Autodesk Fusion 360 part; units mm, degrees
(part 3 of 3)
sketch "Sketch12" plane through (0, 0, 6) normal (0, 0, 1) x (-1, 0, 0)
  line L0 (-92.4617, 84.1384) -> (-86.7336, 92.5805)
  line L1 (-86.7336, 92.5805) -> (-82.7739, 89.3746)
  line L2 (-82.7739, 89.3746) -> (-92.4617, 84.1384)
  line L3 (-84.0126, 80.6229) -> (-80.1679, 87.2648)
  line L4 (-80.1679, 87.2648) -> (-76.1584, 84.0186)
  line L5 (-76.1584, 84.0186) -> (-84.0126, 80.6229)
  line L6 (-75.564, 76.5813) -> (-73.4538, 81.829)
  line L7 (-73.4538, 81.829) -> (-68.7023, 77.9821)
  line L8 (-68.7023, 77.9821) -> (-75.564, 76.5813)
  line L9 (-66.0187, 71.228) -> (-65.6021, 75.4722)
  line L10 (-65.6021, 75.4722) -> (-60.6844, 71.4907)
  line L11 (-60.6844, 71.4907) -> (-66.0187, 71.228)
  line L12 (-49.5335, 59.4079) -> (-45.3919, 59.1098)
  line L13 (-45.3919, 59.1098) -> (-45.0146, 55.4505)
  spline S0 degree 3 poles (-45.0146, 55.4505) (-46.4903, 56.8) (-47.9962, 58.1195) (-49.5335, 59.4079) knots 0.296583 0.296583 0.296583 0.296583 0.351349 0.351349 0.351349 0.351349
  line L14 (-37.9212, 53.0614) -> (-37.9212, 51.766)
  line L15 (-37.9212, 51.766) -> (-37.9212, 48.4975)
  spline S1 degree 3 poles (-37.9212, 48.4975) (-39.1883, 49.8271) (-40.4796, 51.1327) (-41.7959, 52.4137) knots 0.205807 0.205807 0.205807 0.205807 0.256159 0.256159 0.256159 0.256159
  line L16 (-41.7959, 52.4137) -> (-37.9212, 53.0614)
  line L17 (-35.1263, 45.4835) -> (-30.3557, 46.9362)
  line L18 (-30.3557, 46.9362) -> (-32.0809, 42.0059)
  spline S2 degree 3 poles (-32.0809, 42.0059) (-33.0798, 43.1811) (-34.0948, 44.3405) (-35.1263, 45.4835) knots 0.126094 0.126094 0.126094 0.126094 0.168261 0.168261 0.168261 0.168261
  spline S3 degree 3 poles (-26.1093, 34.5476) (-27.3076, 36.135) (-28.5305, 37.698) (-29.7792, 39.2354) knots 0.039267 0.039267 0.039267 0.039267 0.093303 0.093303 0.093303 0.093303
  line L19 (-29.7792, 39.2354) -> (-23.1969, 41.1404)
  line L20 (-23.1969, 41.1404) -> (-26.1093, 34.5476)
  line L21 (-27.7829, 47.0202) -> (-22.7358, 48.9312)
  line L22 (-22.7358, 48.9312) -> (-23.5672, 43.6191)
  line L23 (-23.5672, 43.6191) -> (-27.7829, 47.0202)
  line L24 (-35.0824, 52.9091) -> (-30.8262, 53.9269)
  line L25 (-30.8262, 53.9269) -> (-30.8262, 49.4754)
  line L26 (-30.8262, 49.4754) -> (-35.0824, 52.9091)
  line L27 (-42.6724, 59.0324) -> (-38.5427, 59.1325)
  line L28 (-38.5427, 59.1325) -> (-38.3359, 55.5339)
  line L29 (-38.3359, 55.5339) -> (-42.6724, 59.0324)
  line L30 (-53.3931, 70.682) -> (-57.6141, 71.0867)
  line L31 (-57.6141, 71.0867) -> (-58.1695, 74.9342)
  spline S4 degree 3 poles (-58.1695, 74.9342) (-57.6496, 74.4545) (-57.1267, 73.9777) (-56.6007, 73.5039) (-55.5434, 72.5513) (-54.4741, 71.6108) (-53.3931, 70.682) knots -0.519753 -0.519753 -0.519753 -0.519753 -0.5 -0.5 -0.5 -0.460292 -0.460292 -0.460292 -0.460292
  line L32 (-61.6594, 78.2411) -> (-66.3286, 78.1172)
  line L33 (-66.3286, 78.1172) -> (-66.0088, 82.615)
  spline S5 degree 3 poles (-66.0088, 82.615) (-64.5832, 81.1337) (-63.1337, 79.6754) (-61.6594, 78.2411) knots -0.622035 -0.622035 -0.622035 -0.622035 -0.564532 -0.564532 -0.564532 -0.564532
  line L34 (-68.7436, 85.5164) -> (-73.8681, 84.1998)
  line L35 (-73.8681, 84.1998) -> (-72.3108, 89.4858)
  spline S6 degree 3 poles (-72.3108, 89.4858) (-71.1388, 88.1462) (-69.95, 86.8228) (-68.7436, 85.5164) knots -0.708932 -0.708932 -0.708932 -0.708932 -0.659206 -0.659206 -0.659206 -0.659206
  line L36 (-74.6324, 92.1865) -> (-80.4342, 89.497)
  line L37 (-80.4342, 89.497) -> (-77.8281, 96.0622)
  spline S7 degree 3 poles (-77.8281, 96.0622) (-76.7771, 94.7566) (-75.7121, 93.4645) (-74.6324, 92.1865) knots -0.788777 -0.788777 -0.788777 -0.788777 -0.742083 -0.742083 -0.742083 -0.742083
  line L38 (-85.6123, 93.6745) -> (-78.9776, 97.5027)
  line L39 (-78.9776, 97.5027) -> (-81.7381, 90.5489)
  line L40 (-81.7381, 90.5489) -> (-85.6123, 93.6745)
  line L41 (-79.0459, 88.377) -> (-73.5557, 90.9221)
  line L42 (-73.5557, 90.9221) -> (-75.2158, 85.2871)
  line L43 (-75.2158, 85.2871) -> (-79.0459, 88.377)
  line L44 (-72.3151, 82.9469) -> (-67.5013, 84.1835)
  line L45 (-67.5013, 84.1835) -> (-67.8456, 79.3411)
  line L46 (-67.8456, 79.3411) -> (-72.3151, 82.9469)
  line L47 (-64.4078, 76.5676) -> (-60.0386, 76.6835)
  line L48 (-60.0386, 76.6835) -> (-59.4437, 72.5628)
  line L49 (-59.4437, 72.5628) -> (-64.4078, 76.5676)
  spline S8 degree 3 poles (-45.0116, 63.8871) (-43.5935, 62.8013) (-42.1585, 61.7326) (-40.7069, 60.6805) knots -0.360336 -0.360336 -0.360336 -0.360336 -0.310857 -0.310857 -0.310857 -0.310857
  line L50 (-40.7069, 60.6805) -> (-44.5984, 60.5862)
  line L51 (-44.5984, 60.5862) -> (-45.0116, 63.8871)
  line L52 (-32.6725, 55.1305) -> (-36.6553, 54.1781)
  line L53 (-36.6553, 54.1781) -> (-36.873, 57.9658)
  spline S9 degree 3 poles (-36.873, 57.9658) (-35.4867, 57.0067) (-34.0863, 56.0618) (-32.6725, 55.1305) knots -0.267714 -0.267714 -0.267714 -0.267714 -0.221358 -0.221358 -0.221358 -0.221358
  line L54 (-24.4898, 49.9779) -> (-29.2262, 48.1845)
  line L55 (-29.2262, 48.1845) -> (-29.2262, 52.9038)
  spline S10 degree 3 poles (-29.2262, 52.9038) (-27.6627, 51.913) (-26.0837, 50.9379) (-24.4898, 49.9779) knots -0.183976 -0.183976 -0.183976 -0.183976 -0.133479 -0.133479 -0.133479 -0.133479
  line L56 (-15.7266, 44.9303) -> (-22.1293, 42.4591)
  line L57 (-22.1293, 42.4591) -> (-21.2525, 48.0608)
  spline S11 degree 3 poles (-21.2525, 48.0608) (-19.8324, 47.2338) (-18.401, 46.4181) (-16.9588, 45.6135) (-16.549, 45.3849) (-16.1382, 45.1571) (-15.7266, 44.9303) knots -0.099506 -0.099506 -0.099506 -0.099506 -0.055069 -0.055069 -0.055069 -0.042441 -0.042441 -0.042441 -0.042441
  line L58 (-30.8842, 40.5813) -> (-29.0347, 45.8668)
  line L59 (-29.0347, 45.8668) -> (-24.7124, 42.3674)
  line L60 (-24.7124, 42.3674) -> (-30.8842, 40.5813)
  line L61 (-36.3212, 46.7922) -> (-36.3212, 51.766)
  line L62 (-36.3212, 51.766) -> (-31.8569, 48.1516)
  line L63 (-31.8569, 48.1516) -> (-36.3212, 46.7922)
  line L64 (-43.2354, 53.7952) -> (-43.6369, 57.6889)
  line L65 (-43.6369, 57.6889) -> (-39.5819, 54.4059)
  line L66 (-39.5819, 54.4059) -> (-43.2354, 53.7952)
  line L67 (-63.64, 69.7432) -> (-58.8192, 69.9806)
  line L68 (-58.8192, 69.9806) -> (-58.101, 66.0186)
  spline S12 degree 3 poles (-58.101, 66.0186) (-59.9089, 67.2995) (-61.7555, 68.5409) (-63.64, 69.7432) knots 0.44941 0.44941 0.44941 0.44941 0.509295 0.509295 0.509295 0.509295
  line L69 (-73.3235, 75.4057) -> (-67.0915, 76.678)
  line L70 (-67.0915, 76.678) -> (-67.5366, 72.1422)
  spline S13 degree 3 poles (-67.5366, 72.1422) (-69.4303, 73.2669) (-71.3596, 74.3545) (-73.3235, 75.4057) knots 0.550019 0.550019 0.550019 0.550019 0.608612 0.608612 0.608612 0.608612
  line L71 (-82.0425, 79.7315) -> (-74.7548, 82.8823)
  line L72 (-74.7548, 82.8823) -> (-76.996, 77.3086)
  spline S14 degree 3 poles (-76.996, 77.3086) (-77.9206, 77.7723) (-78.8524, 78.2283) (-79.7914, 78.6767) (-80.5375, 79.0329) (-81.2878, 79.3845) (-82.0425, 79.7315) knots 0.644744 0.644744 0.644744 0.644744 0.671746 0.671746 0.671746 0.693198 0.693198 0.693198 0.693198
  line L73 (-90.517, 83.3708) -> (-81.4267, 88.284)
  line L74 (-81.4267, 88.284) -> (-85.4862, 81.271)
  spline S15 degree 3 poles (-85.4862, 81.271) (-87.1438, 81.9913) (-88.821, 82.691) (-90.517, 83.3708) knots 0.725554 0.725554 0.725554 0.725554 0.77189 0.77189 0.77189 0.77189
  spline S16 degree 3 poles (-93.9955, 84.7275) (-96.255, 85.585) (-98.5463, 86.4092) (-100.8677, 87.202) knots 0.803334 0.803334 0.803334 0.803334 0.864159 0.864159 0.864159 0.864159
  line L75 (-100.8677, 87.202) -> (-87.9816, 93.5909)
  line L76 (-87.9816, 93.5909) -> (-93.9955, 84.7275)
  line L77 (22.7358, 48.9312) -> (27.7829, 47.0202)
  line L78 (27.7829, 47.0202) -> (23.5672, 43.6191)
  line L79 (23.5672, 43.6191) -> (22.7358, 48.9312)
  line L80 (30.8262, 53.9269) -> (35.0824, 52.9091)
  line L81 (35.0824, 52.9091) -> (30.8262, 49.4754)
  line L82 (30.8262, 49.4754) -> (30.8262, 53.9269)
  line L83 (38.5427, 59.1325) -> (42.6724, 59.0324)
  line L84 (42.6724, 59.0324) -> (38.3359, 55.5339)
  line L85 (38.3359, 55.5339) -> (38.5427, 59.1325)
  spline S17 degree 3 poles (53.3931, 70.682) (54.4741, 71.6108) (55.5434, 72.5513) (56.6007, 73.5039) (57.1267, 73.9777) (57.6496, 74.4545) (58.1695, 74.9342) knots 0.460292 0.460292 0.460292 0.460292 0.5 0.5 0.5 0.519753 0.519753 0.519753 0.519753
  line L86 (58.1695, 74.9342) -> (57.6141, 71.0867)
  line L87 (57.6141, 71.0867) -> (53.3931, 70.682)
  line L88 (66.0088, 82.615) -> (66.3286, 78.1172)
  line L89 (66.3286, 78.1172) -> (61.6594, 78.2411)
  spline S18 degree 3 poles (61.6594, 78.2411) (63.1337, 79.6754) (64.5832, 81.1337) (66.0088, 82.615) knots 0.564532 0.564532 0.564532 0.564532 0.622035 0.622035 0.622035 0.622035
  line L90 (72.3108, 89.4858) -> (73.8681, 84.1998)
  line L91 (73.8681, 84.1998) -> (68.7436, 85.5164)
  spline S19 degree 3 poles (68.7436, 85.5164) (69.95, 86.8228) (71.1388, 88.1462) (72.3108, 89.4858) knots 0.659206 0.659206 0.659206 0.659206 0.708932 0.708932 0.708932 0.708932
  spline S20 degree 3 poles (74.6324, 92.1865) (75.7121, 93.4645) (76.7771, 94.7566) (77.8281, 96.0622) knots 0.742083 0.742083 0.742083 0.742083 0.788777 0.788777 0.788777 0.788777
  line L92 (77.8281, 96.0622) -> (80.4342, 89.497)
  line L93 (80.4342, 89.497) -> (74.6324, 92.1865)
  line L94 (86.9472, 94.7515) -> (79.9758, 98.774)
  spline S21 degree 3 poles (79.9758, 98.774) (81.2999, 100.473) (82.6013, 102.1938) (83.881, 103.9354) knots 0.820879 0.820879 0.820879 0.820879 0.880798 0.880798 0.880798 0.880798
  line L95 (86.7336, 92.5805) -> (92.4617, 84.1384)
  line L96 (92.4617, 84.1384) -> (82.7739, 89.3746)
  line L97 (82.7739, 89.3746) -> (86.7336, 92.5805)
  line L98 (80.1679, 87.2648) -> (84.0126, 80.6229)
  line L99 (84.0126, 80.6229) -> (76.1584, 84.0186)
  line L100 (76.1584, 84.0186) -> (80.1679, 87.2648)
  line L101 (73.4538, 81.829) -> (75.564, 76.5813)
  line L102 (75.564, 76.5813) -> (68.7023, 77.9821)
  line L103 (68.7023, 77.9821) -> (73.4538, 81.829)
  line L104 (65.6021, 75.4722) -> (66.0187, 71.228)
  line L105 (66.0187, 71.228) -> (60.6844, 71.4907)
  line L106 (60.6844, 71.4907) -> (65.6021, 75.4722)
  line L107 (45.3919, 59.1098) -> (49.5335, 59.4079)
  spline S22 degree 3 poles (49.5335, 59.4079) (47.9962, 58.1195) (46.4903, 56.8) (45.0146, 55.4505) knots -0.351349 -0.351349 -0.351349 -0.351349 -0.296583 -0.296583 -0.296583 -0.296583
  line L108 (45.0146, 55.4505) -> (45.3919, 59.1098)
  line L109 (37.9212, 53.0614) -> (41.7959, 52.4137)
  spline S23 degree 3 poles (41.7959, 52.4137) (40.4796, 51.1327) (39.1883, 49.8271) (37.9212, 48.4975) knots -0.256159 -0.256159 -0.256159 -0.256159 -0.205807 -0.205807 -0.205807 -0.205807
  line L110 (37.9212, 48.4975) -> (37.9212, 51.766)
  line L111 (37.9212, 51.766) -> (37.9212, 53.0614)
  line L112 (30.3557, 46.9362) -> (35.1263, 45.4835)
  spline S24 degree 3 poles (35.1263, 45.4835) (34.0948, 44.3405) (33.0798, 43.1811) (32.0809, 42.0059) knots -0.168261 -0.168261 -0.168261 -0.168261 -0.126094 -0.126094 -0.126094 -0.126094
  line L113 (32.0809, 42.0059) -> (30.3557, 46.9362)
  spline S25 degree 3 poles (29.7792, 39.2354) (28.5305, 37.698) (27.3076, 36.135) (26.1093, 34.5476) knots -0.093303 -0.093303 -0.093303 -0.093303 -0.039267 -0.039267 -0.039267 -0.039267
  line L114 (26.1093, 34.5476) -> (23.1969, 41.1404)
  line L115 (23.1969, 41.1404) -> (29.7792, 39.2354)
  line L116 (29.0347, 45.8668) -> (30.8842, 40.5813)
  line L117 (30.8842, 40.5813) -> (24.7124, 42.3674)
  line L118 (24.7124, 42.3674) -> (29.0347, 45.8668)
  line L119 (36.3212, 51.766) -> (36.3212, 46.7922)
  line L120 (36.3212, 46.7922) -> (31.8569, 48.1516)
  line L121 (31.8569, 48.1516) -> (36.3212, 51.766)
  line L122 (43.6369, 57.6889) -> (43.2354, 53.7952)
  line L123 (43.2354, 53.7952) -> (39.5819, 54.4059)
  line L124 (39.5819, 54.4059) -> (43.6369, 57.6889)
  line L125 (58.8192, 69.9806) -> (63.64, 69.7432)
  spline S26 degree 3 poles (63.64, 69.7432) (61.7555, 68.5409) (59.9089, 67.2995) (58.101, 66.0186) knots -0.509295 -0.509295 -0.509295 -0.509295 -0.44941 -0.44941 -0.44941 -0.44941
  line L126 (58.101, 66.0186) -> (58.8192, 69.9806)
  line L127 (67.0915, 76.678) -> (73.3235, 75.4057)
  spline S27 degree 3 poles (73.3235, 75.4057) (71.3596, 74.3545) (69.4303, 73.2669) (67.5366, 72.1422) knots -0.608612 -0.608612 -0.608612 -0.608612 -0.550019 -0.550019 -0.550019 -0.550019
  line L128 (67.5366, 72.1422) -> (67.0915, 76.678)
  line L129 (74.7548, 82.8823) -> (82.0425, 79.7315)
  spline S28 degree 3 poles (82.0425, 79.7315) (81.2878, 79.3845) (80.5375, 79.0329) (79.7914, 78.6767) (78.8524, 78.2283) (77.9206, 77.7723) (76.996, 77.3086) knots -0.693198 -0.693198 -0.693198 -0.693198 -0.671746 -0.671746 -0.671746 -0.644744 -0.644744 -0.644744 -0.644744
  line L130 (76.996, 77.3086) -> (74.7548, 82.8823)
  spline S29 degree 3 poles (90.517, 83.3708) (88.821, 82.691) (87.1438, 81.9913) (85.4862, 81.271) knots -0.77189 -0.77189 -0.77189 -0.77189 -0.725554 -0.725554 -0.725554 -0.725554
  line L131 (85.4862, 81.271) -> (81.4267, 88.284)
  line L132 (81.4267, 88.284) -> (90.517, 83.3708)
  spline S30 degree 3 poles (100.8677, 87.202) (98.5463, 86.4092) (96.255, 85.585) (93.9955, 84.7275) knots -0.864159 -0.864159 -0.864159 -0.864159 -0.803334 -0.803334 -0.803334 -0.803334
  line L133 (93.9955, 84.7275) -> (87.9816, 93.5909)
  line L134 (87.9816, 93.5909) -> (100.8677, 87.202)
  line L135 (78.9776, 97.5027) -> (85.6123, 93.6745)
  line L136 (85.6123, 93.6745) -> (81.7381, 90.5489)
  line L137 (81.7381, 90.5489) -> (78.9776, 97.5027)
  line L138 (73.5557, 90.9221) -> (79.0459, 88.377)
  line L139 (79.0459, 88.377) -> (75.2158, 85.2871)
  line L140 (75.2158, 85.2871) -> (73.5557, 90.9221)
  line L141 (67.5013, 84.1835) -> (72.3151, 82.9469)
  line L142 (72.3151, 82.9469) -> (67.8456, 79.3411)
  line L143 (67.8456, 79.3411) -> (67.5013, 84.1835)
  line L144 (60.0386, 76.6835) -> (64.4078, 76.5676)
  line L145 (64.4078, 76.5676) -> (59.4437, 72.5628)
  line L146 (59.4437, 72.5628) -> (60.0386, 76.6835)
  spline S31 degree 3 poles (40.7069, 60.6805) (42.1585, 61.7326) (43.5935, 62.8013) (45.0116, 63.8871) knots 0.310857 0.310857 0.310857 0.310857 0.360336 0.360336 0.360336 0.360336
  line L147 (45.0116, 63.8871) -> (44.5984, 60.5862)
  line L148 (44.5984, 60.5862) -> (40.7069, 60.6805)
  spline S32 degree 3 poles (32.6725, 55.1305) (34.0863, 56.0618) (35.4867, 57.0067) (36.873, 57.9658) knots 0.221358 0.221358 0.221358 0.221358 0.267714 0.267714 0.267714 0.267714
  line L149 (36.873, 57.9658) -> (36.6553, 54.1781)
  line L150 (36.6553, 54.1781) -> (32.6725, 55.1305)
  spline S33 degree 3 poles (24.4898, 49.9779) (26.0837, 50.9379) (27.6627, 51.913) (29.2262, 52.9038) knots 0.133479 0.133479 0.133479 0.133479 0.183976 0.183976 0.183976 0.183976
  line L151 (29.2262, 52.9038) -> (29.2262, 48.1845)
  line L152 (29.2262, 48.1845) -> (24.4898, 49.9779)
  spline S34 degree 3 poles (15.7266, 44.9303) (16.1382, 45.1571) (16.549, 45.3849) (16.9588, 45.6135) (18.401, 46.4181) (19.8324, 47.2338) (21.2525, 48.0608) knots 0.042441 0.042441 0.042441 0.042441 0.055069 0.055069 0.055069 0.099506 0.099506 0.099506 0.099506
  line L153 (21.2525, 48.0608) -> (22.1293, 42.4591)
  line L154 (22.1293, 42.4591) -> (15.7266, 44.9303)
  arc A0 (23.3348, 9) -> (22.3348, 10) centre (22.3348, 9) ccw
  line L155 (23.3348, 9) -> (23.3348, -9)
  arc A1 (22.3348, -10) -> (23.3348, -9) centre (22.3348, -9) ccw
  line L156 (22.3348, -10) -> (21.8348, -10)
  arc A2 (20.8348, -9) -> (21.8348, -10) centre (21.8348, -9) ccw
  line L157 (20.8348, -9) -> (20.8348, 9)
  arc A3 (21.8348, 10) -> (20.8348, 9) centre (21.8348, 9) ccw
  line L158 (21.8348, 10) -> (22.3348, 10)
  arc A4 (-23.3348, -9) -> (-22.3348, -10) centre (-22.3348, -9) ccw
  line L159 (-23.3348, -9) -> (-23.3348, 9)
  arc A5 (-22.3348, 10) -> (-23.3348, 9) centre (-22.3348, 9) ccw
  line L160 (-22.3348, 10) -> (-21.8348, 10)
  arc A6 (-20.8348, 9) -> (-21.8348, 10) centre (-21.8348, 9) ccw
  line L161 (-20.8348, 9) -> (-20.8348, -9)
  arc A7 (-21.8348, -10) -> (-20.8348, -9) centre (-21.8348, -9) ccw
  line L162 (-21.8348, -10) -> (-22.3348, -10)
  line L163 (30.8842, -40.5813) -> (29.0347, -45.8668)
  line L164 (29.0347, -45.8668) -> (24.7124, -42.3674)
  line L165 (24.7124, -42.3674) -> (30.8842, -40.5813)
  line L166 (36.3212, -46.7922) -> (36.3212, -51.766)
  line L167 (36.3212, -51.766) -> (31.8569, -48.1516)
  line L168 (31.8569, -48.1516) -> (36.3212, -46.7922)
  line L169 (42.6724, -59.0324) -> (38.5427, -59.1325)
  line L170 (38.5427, -59.1325) -> (38.3359, -55.5339)
  line L171 (38.3359, -55.5339) -> (42.6724, -59.0324)
  line L172 (49.5335, -59.4079) -> (45.3919, -59.1098)
  line L173 (45.3919, -59.1098) -> (45.0146, -55.4505)
  spline S35 degree 3 poles (45.0146, -55.4505) (46.4903, -56.8) (47.9962, -58.1195) (49.5335, -59.4079) knots 0.296583 0.296583 0.296583 0.296583 0.351349 0.351349 0.351349 0.351349
  line L174 (37.9212, -53.0614) -> (37.9212, -51.766)
  line L175 (37.9212, -51.766) -> (37.9212, -48.4975)
  spline S36 degree 3 poles (37.9212, -48.4975) (39.1883, -49.8271) (40.4796, -51.1327) (41.7959, -52.4137) knots 0.205807 0.205807 0.205807 0.205807 0.256159 0.256159 0.256159 0.256159
  line L176 (41.7959, -52.4137) -> (37.9212, -53.0614)
  line L177 (35.1263, -45.4835) -> (30.3557, -46.9362)
  line L178 (30.3557, -46.9362) -> (32.0809, -42.0059)
  spline S37 degree 3 poles (32.0809, -42.0059) (33.0798, -43.1811) (34.0948, -44.3405) (35.1263, -45.4835) knots 0.126094 0.126094 0.126094 0.126094 0.168261 0.168261 0.168261 0.168261
  spline S38 degree 3 poles (26.1093, -34.5476) (27.3076, -36.135) (28.5305, -37.698) (29.7792, -39.2354) knots 0.039267 0.039267 0.039267 0.039267 0.093303 0.093303 0.093303 0.093303
  line L179 (29.7792, -39.2354) -> (23.1969, -41.1404)
  line L180 (23.1969, -41.1404) -> (26.1093, -34.5476)
  line L181 (27.7829, -47.0202) -> (22.7358, -48.9312)
  line L182 (22.7358, -48.9312) -> (23.5672, -43.6191)
  line L183 (23.5672, -43.6191) -> (27.7829, -47.0202)
  line L184 (35.0824, -52.9091) -> (30.8262, -53.9269)
  line L185 (30.8262, -53.9269) -> (30.8262, -49.4754)
  line L186 (30.8262, -49.4754) -> (35.0824, -52.9091)
  line L187 (43.2354, -53.7952) -> (43.6369, -57.6889)
  line L188 (43.6369, -57.6889) -> (39.5819, -54.4059)
  line L189 (39.5819, -54.4059) -> (43.2354, -53.7952)
  spline S39 degree 3 poles (45.0116, -63.8871) (43.5935, -62.8013) (42.1585, -61.7326) (40.7069, -60.6805) knots -0.360336 -0.360336 -0.360336 -0.360336 -0.310857 -0.310857 -0.310857 -0.310857
  line L190 (40.7069, -60.6805) -> (44.5984, -60.5862)
  line L191 (44.5984, -60.5862) -> (45.0116, -63.8871)
  line L192 (36.6553, -54.1781) -> (36.873, -57.9658)
  spline S40 degree 3 poles (36.873, -57.9658) (35.4867, -57.0067) (34.0863, -56.0618) (32.6725, -55.1305) knots -0.267714 -0.267714 -0.267714 -0.267714 -0.221358 -0.221358 -0.221358 -0.221358
  line L193 (32.6725, -55.1305) -> (36.6553, -54.1781)
  line L194 (29.2262, -48.1845) -> (29.2262, -52.9038)
  spline S41 degree 3 poles (29.2262, -52.9038) (27.6627, -51.913) (26.0837, -50.9379) (24.4898, -49.9779) knots -0.183976 -0.183976 -0.183976 -0.183976 -0.133479 -0.133479 -0.133479 -0.133479
  line L195 (24.4898, -49.9779) -> (29.2262, -48.1845)
  spline S42 degree 3 poles (21.2525, -48.0608) (19.8324, -47.2338) (18.401, -46.4181) (16.9588, -45.6135) (16.549, -45.3849) (16.1382, -45.1571) (15.7266, -44.9303) knots -0.099506 -0.099506 -0.099506 -0.099506 -0.055069 -0.055069 -0.055069 -0.042441 -0.042441 -0.042441 -0.042441
  line L196 (15.7266, -44.9303) -> (22.1293, -42.4591)
  line L197 (22.1293, -42.4591) -> (21.2525, -48.0608)
  line L198 (74.6324, -92.1865) -> (80.4342, -89.497)
  line L199 (80.4342, -89.497) -> (77.8281, -96.0622)
  spline S43 degree 3 poles (77.8281, -96.0622) (76.7771, -94.7566) (75.7121, -93.4645) (74.6324, -92.1865) knots -0.788777 -0.788777 -0.788777 -0.788777 -0.742083 -0.742083 -0.742083 -0.742083
  spline S44 degree 3 poles (66.0088, -82.615) (64.5832, -81.1337) (63.1337, -79.6754) (61.6594, -78.2411) knots -0.622035 -0.622035 -0.622035 -0.622035 -0.564532 -0.564532 -0.564532 -0.564532
  line L200 (61.6594, -78.2411) -> (66.3286, -78.1172)
  line L201 (66.3286, -78.1172) -> (66.0088, -82.615)
  line L202 (66.0187, -71.228) -> (65.6021, -75.4722)
  line L203 (65.6021, -75.4722) -> (60.6844, -71.4907)
  line L204 (60.6844, -71.4907) -> (66.0187, -71.228)
  line L205 (84.0126, -80.6229) -> (80.1679, -87.2648)
  line L206 (80.1679, -87.2648) -> (76.1584, -84.0186)
  line L207 (76.1584, -84.0186) -> (84.0126, -80.6229)
  line L208 (100.8677, -87.202) -> (87.9816, -93.5909)
  line L209 (87.9816, -93.5909) -> (93.9955, -84.7275)
  spline S45 degree 3 poles (93.9955, -84.7275) (96.255, -85.585) (98.5463, -86.4092) (100.8677, -87.202) knots 0.803334 0.803334 0.803334 0.803334 0.864159 0.864159 0.864159 0.864159
  line L210 (82.0425, -79.7315) -> (74.7548, -82.8823)
  line L211 (74.7548, -82.8823) -> (76.996, -77.3086)
  spline S46 degree 3 poles (76.996, -77.3086) (77.9206, -77.7723) (78.8524, -78.2283) (79.7914, -78.6767) (80.5375, -79.0329) (81.2878, -79.3845) (82.0425, -79.7315) knots 0.644744 0.644744 0.644744 0.644744 0.671746 0.671746 0.671746 0.693198 0.693198 0.693198 0.693198
  line L212 (63.64, -69.7432) -> (58.8192, -69.9806)
  line L213 (58.8192, -69.9806) -> (58.101, -66.0186)
  spline S47 degree 3 poles (58.101, -66.0186) (59.9089, -67.2995) (61.7555, -68.5409) (63.64, -69.7432) knots 0.44941 0.44941 0.44941 0.44941 0.509295 0.509295 0.509295 0.509295
  line L214 (72.3151, -82.9469) -> (67.5013, -84.1835)
  line L215 (67.5013, -84.1835) -> (67.8456, -79.3411)
  line L216 (67.8456, -79.3411) -> (72.3151, -82.9469)
  line L217 (85.6123, -93.6745) -> (78.9776, -97.5027)
  line L218 (78.9776, -97.5027) -> (81.7381, -90.5489)
  line L219 (81.7381, -90.5489) -> (85.6123, -93.6745)
  line L220 (79.0459, -88.377) -> (73.5557, -90.9221)
  line L221 (73.5557, -90.9221) -> (75.2158, -85.2871)
  line L222 (75.2158, -85.2871) -> (79.0459, -88.377)
  line L223 (64.4078, -76.5676) -> (60.0386, -76.6835)
  line L224 (60.0386, -76.6835) -> (59.4437, -72.5628)
  line L225 (59.4437, -72.5628) -> (64.4078, -76.5676)
  line L226 (73.3235, -75.4057) -> (67.0915, -76.678)
  line L227 (67.0915, -76.678) -> (67.5366, -72.1422)
  spline S48 degree 3 poles (67.5366, -72.1422) (69.4303, -73.2669) (71.3596, -74.3545) (73.3235, -75.4057) knots 0.550019 0.550019 0.550019 0.550019 0.608612 0.608612 0.608612 0.608612
  line L228 (90.517, -83.3708) -> (81.4267, -88.284)
  line L229 (81.4267, -88.284) -> (85.4862, -81.271)
  spline S49 degree 3 poles (85.4862, -81.271) (87.1438, -81.9913) (88.821, -82.691) (90.517, -83.3708) knots 0.725554 0.725554 0.725554 0.725554 0.77189 0.77189 0.77189 0.77189
  line L230 (92.4617, -84.1384) -> (86.7336, -92.5805)
  line L231 (86.7336, -92.5805) -> (82.7739, -89.3746)
  line L232 (82.7739, -89.3746) -> (92.4617, -84.1384)
  line L233 (75.564, -76.5813) -> (73.4538, -81.829)
  line L234 (73.4538, -81.829) -> (68.7023, -77.9821)
  line L235 (68.7023, -77.9821) -> (75.564, -76.5813)
  spline S50 degree 3 poles (58.1695, -74.9342) (57.6496, -74.4545) (57.1267, -73.9777) (56.6007, -73.5039) (55.5434, -72.5513) (54.4741, -71.6108) (53.3931, -70.682) knots -0.519753 -0.519753 -0.519753 -0.519753 -0.5 -0.5 -0.5 -0.460292 -0.460292 -0.460292 -0.460292
  line L236 (53.3931, -70.682) -> (57.6141, -71.0867)
  line L237 (57.6141, -71.0867) -> (58.1695, -74.9342)
  spline S51 degree 3 poles (72.3108, -89.4858) (71.1388, -88.1462) (69.95, -86.8228) (68.7436, -85.5164) knots -0.708932 -0.708932 -0.708932 -0.708932 -0.659206 -0.659206 -0.659206 -0.659206
  line L238 (68.7436, -85.5164) -> (73.8681, -84.1998)
  line L239 (73.8681, -84.1998) -> (72.3108, -89.4858)
  spline S52 degree 3 poles (83.881, -103.9354) (82.6013, -102.1938) (81.2999, -100.473) (79.9758, -98.774) knots -0.880798 -0.880798 -0.880798 -0.880798 -0.820879 -0.820879 -0.820879 -0.820879
  line L240 (79.9758, -98.774) -> (86.9472, -94.7515)
  line L241 (-60.0386, -76.6835) -> (-64.4078, -76.5676)
  line L242 (-64.4078, -76.5676) -> (-59.4437, -72.5628)
  line L243 (-59.4437, -72.5628) -> (-60.0386, -76.6835)
  line L244 (-67.5013, -84.1835) -> (-72.3151, -82.9469)
  line L245 (-72.3151, -82.9469) -> (-67.8456, -79.3411)
  line L246 (-67.8456, -79.3411) -> (-67.5013, -84.1835)
  line L247 (-73.5557, -90.9221) -> (-79.0459, -88.377)
  line L248 (-79.0459, -88.377) -> (-75.2158, -85.2871)
  line L249 (-75.2158, -85.2871) -> (-73.5557, -90.9221)
  spline S53 degree 3 poles (-79.9758, -98.774) (-81.2999, -100.473) (-82.6013, -102.1938) (-83.881, -103.9354) knots 0.820879 0.820879 0.820879 0.820879 0.880798 0.880798 0.880798 0.880798
  line L250 (-86.9472, -94.7515) -> (-79.9758, -98.774)
  spline S54 degree 3 poles (-100.8677, -87.202) (-98.5463, -86.4092) (-96.255, -85.585) (-93.9955, -84.7275) knots -0.864159 -0.864159 -0.864159 -0.864159 -0.803334 -0.803334 -0.803334 -0.803334
  line L251 (-93.9955, -84.7275) -> (-87.9816, -93.5909)
  line L252 (-87.9816, -93.5909) -> (-100.8677, -87.202)
  line L253 (-78.9776, -97.5027) -> (-85.6123, -93.6745)
  line L254 (-85.6123, -93.6745) -> (-81.7381, -90.5489)
  line L255 (-81.7381, -90.5489) -> (-78.9776, -97.5027)
  line L256 (-74.7548, -82.8823) -> (-82.0425, -79.7315)
  spline S55 degree 3 poles (-82.0425, -79.7315) (-81.2878, -79.3845) (-80.5375, -79.0329) (-79.7914, -78.6767) (-78.8524, -78.2283) (-77.9206, -77.7723) (-76.996, -77.3086) knots -0.693198 -0.693198 -0.693198 -0.693198 -0.671746 -0.671746 -0.671746 -0.644744 -0.644744 -0.644744 -0.644744
  line L257 (-76.996, -77.3086) -> (-74.7548, -82.8823)
  line L258 (-67.0915, -76.678) -> (-73.3235, -75.4057)
  spline S56 degree 3 poles (-73.3235, -75.4057) (-71.3596, -74.3545) (-69.4303, -73.2669) (-67.5366, -72.1422) knots -0.608612 -0.608612 -0.608612 -0.608612 -0.550019 -0.550019 -0.550019 -0.550019
  line L259 (-67.5366, -72.1422) -> (-67.0915, -76.678)
  line L260 (-58.8192, -69.9806) -> (-63.64, -69.7432)
  spline S57 degree 3 poles (-63.64, -69.7432) (-61.7555, -68.5409) (-59.9089, -67.2995) (-58.101, -66.0186) knots -0.509295 -0.509295 -0.509295 -0.509295 -0.44941 -0.44941 -0.44941 -0.44941
  line L261 (-58.101, -66.0186) -> (-58.8192, -69.9806)
  line L262 (-65.6021, -75.4722) -> (-66.0187, -71.228)
  line L263 (-66.0187, -71.228) -> (-60.6844, -71.4907)
  line L264 (-60.6844, -71.4907) -> (-65.6021, -75.4722)
  line L265 (-73.4538, -81.829) -> (-75.564, -76.5813)
  line L266 (-75.564, -76.5813) -> (-68.7023, -77.9821)
  line L267 (-68.7023, -77.9821) -> (-73.4538, -81.829)
  line L268 (-80.1679, -87.2648) -> (-84.0126, -80.6229)
  line L269 (-84.0126, -80.6229) -> (-76.1584, -84.0186)
  line L270 (-76.1584, -84.0186) -> (-80.1679, -87.2648)
  spline S58 degree 3 poles (-90.517, -83.3708) (-88.821, -82.691) (-87.1438, -81.9913) (-85.4862, -81.271) knots -0.77189 -0.77189 -0.77189 -0.77189 -0.725554 -0.725554 -0.725554 -0.725554
  line L271 (-85.4862, -81.271) -> (-81.4267, -88.284)
  line L272 (-81.4267, -88.284) -> (-90.517, -83.3708)
  line L273 (-86.7336, -92.5805) -> (-92.4617, -84.1384)
  line L274 (-92.4617, -84.1384) -> (-82.7739, -89.3746)
  line L275 (-82.7739, -89.3746) -> (-86.7336, -92.5805)
  spline S59 degree 3 poles (-74.6324, -92.1865) (-75.7121, -93.4645) (-76.7771, -94.7566) (-77.8281, -96.0622) knots 0.742083 0.742083 0.742083 0.742083 0.788777 0.788777 0.788777 0.788777
  line L276 (-77.8281, -96.0622) -> (-80.4342, -89.497)
  line L277 (-80.4342, -89.497) -> (-74.6324, -92.1865)
  spline S60 degree 3 poles (-68.7436, -85.5164) (-69.95, -86.8228) (-71.1388, -88.1462) (-72.3108, -89.4858) knots 0.659206 0.659206 0.659206 0.659206 0.708932 0.708932 0.708932 0.708932
  line L278 (-72.3108, -89.4858) -> (-73.8681, -84.1998)
  line L279 (-73.8681, -84.1998) -> (-68.7436, -85.5164)
  spline S61 degree 3 poles (-61.6594, -78.2411) (-63.1337, -79.6754) (-64.5832, -81.1337) (-66.0088, -82.615) knots 0.564532 0.564532 0.564532 0.564532 0.622035 0.622035 0.622035 0.622035
  line L280 (-66.0088, -82.615) -> (-66.3286, -78.1172)
  line L281 (-66.3286, -78.1172) -> (-61.6594, -78.2411)
  spline S62 degree 3 poles (-53.3931, -70.682) (-54.4741, -71.6108) (-55.5434, -72.5513) (-56.6007, -73.5039) (-57.1267, -73.9777) (-57.6496, -74.4545) (-58.1695, -74.9342) knots 0.460292 0.460292 0.460292 0.460292 0.5 0.5 0.5 0.519753 0.519753 0.519753 0.519753
  line L282 (-58.1695, -74.9342) -> (-57.6141, -71.0867)
  line L283 (-57.6141, -71.0867) -> (-53.3931, -70.682)
  line L284 (-30.3557, -46.9362) -> (-35.1263, -45.4835)
  spline S63 degree 3 poles (-35.1263, -45.4835) (-34.0948, -44.3405) (-33.0798, -43.1811) (-32.0809, -42.0059) knots -0.168261 -0.168261 -0.168261 -0.168261 -0.126094 -0.126094 -0.126094 -0.126094
  line L285 (-32.0809, -42.0059) -> (-30.3557, -46.9362)
  line L286 (-45.3919, -59.1098) -> (-49.5335, -59.4079)
  spline S64 degree 3 poles (-49.5335, -59.4079) (-47.9962, -58.1195) (-46.4903, -56.8) (-45.0146, -55.4505) knots -0.351349 -0.351349 -0.351349 -0.351349 -0.296583 -0.296583 -0.296583 -0.296583
  line L287 (-45.0146, -55.4505) -> (-45.3919, -59.1098)
  line L288 (-30.8262, -53.9269) -> (-35.0824, -52.9091)
  line L289 (-35.0824, -52.9091) -> (-30.8262, -49.4754)
  line L290 (-30.8262, -49.4754) -> (-30.8262, -53.9269)
  spline S65 degree 3 poles (-15.7266, -44.9303) (-16.1382, -45.1571) (-16.549, -45.3849) (-16.9588, -45.6135) (-18.401, -46.4181) (-19.8324, -47.2338) (-21.2525, -48.0608) knots 0.042441 0.042441 0.042441 0.042441 0.055069 0.055069 0.055069 0.099506 0.099506 0.099506 0.099506
  line L291 (-21.2525, -48.0608) -> (-22.1293, -42.4591)
  line L292 (-22.1293, -42.4591) -> (-15.7266, -44.9303)
  spline S66 degree 3 poles (-32.6725, -55.1305) (-34.0863, -56.0618) (-35.4867, -57.0067) (-36.873, -57.9658) knots 0.221358 0.221358 0.221358 0.221358 0.267714 0.267714 0.267714 0.267714
  line L293 (-36.873, -57.9658) -> (-36.6553, -54.1781)
  line L294 (-36.6553, -54.1781) -> (-32.6725, -55.1305)
  line L295 (-43.6369, -57.6889) -> (-43.2354, -53.7952)
  line L296 (-43.2354, -53.7952) -> (-39.5819, -54.4059)
  line L297 (-39.5819, -54.4059) -> (-43.6369, -57.6889)
  line L298 (-29.0347, -45.8668) -> (-30.8842, -40.5813)
  line L299 (-30.8842, -40.5813) -> (-24.7124, -42.3674)
  line L300 (-24.7124, -42.3674) -> (-29.0347, -45.8668)
  line L301 (-36.3212, -51.766) -> (-36.3212, -46.7922)
  line L302 (-36.3212, -46.7922) -> (-31.8569, -48.1516)
  line L303 (-31.8569, -48.1516) -> (-36.3212, -51.766)
  spline S67 degree 3 poles (-40.7069, -60.6805) (-42.1585, -61.7326) (-43.5935, -62.8013) (-45.0116, -63.8871) knots 0.310857 0.310857 0.310857 0.310857 0.360336 0.360336 0.360336 0.360336
  line L304 (-45.0116, -63.8871) -> (-44.5984, -60.5862)
  line L305 (-44.5984, -60.5862) -> (-40.7069, -60.6805)
  spline S68 degree 3 poles (-24.4898, -49.9779) (-26.0837, -50.9379) (-27.6627, -51.913) (-29.2262, -52.9038) knots 0.133479 0.133479 0.133479 0.133479 0.183976 0.183976 0.183976 0.183976
  line L306 (-29.2262, -52.9038) -> (-29.2262, -48.1845)
  line L307 (-29.2262, -48.1845) -> (-24.4898, -49.9779)
  line L308 (-22.7358, -48.9312) -> (-27.7829, -47.0202)
  line L309 (-27.7829, -47.0202) -> (-23.5672, -43.6191)
  line L310 (-23.5672, -43.6191) -> (-22.7358, -48.9312)
  line L311 (-38.5427, -59.1325) -> (-42.6724, -59.0324)
  line L312 (-42.6724, -59.0324) -> (-38.3359, -55.5339)
  line L313 (-38.3359, -55.5339) -> (-38.5427, -59.1325)
  line L314 (-37.9212, -53.0614) -> (-41.7959, -52.4137)
  spline S69 degree 3 poles (-41.7959, -52.4137) (-40.4796, -51.1327) (-39.1883, -49.8271) (-37.9212, -48.4975) knots -0.256159 -0.256159 -0.256159 -0.256159 -0.205807 -0.205807 -0.205807 -0.205807
  line L315 (-37.9212, -48.4975) -> (-37.9212, -51.766)
  line L316 (-37.9212, -51.766) -> (-37.9212, -53.0614)
  line L317 (-23.1969, -41.1404) -> (-29.7792, -39.2354)
  spline S70 degree 3 poles (-29.7792, -39.2354) (-28.5305, -37.698) (-27.3076, -36.135) (-26.1093, -34.5476) knots -0.093303 -0.093303 -0.093303 -0.093303 -0.039267 -0.039267 -0.039267 -0.039267
  line L318 (-26.1093, -34.5476) -> (-23.1969, -41.1404)
  line L319 (-10, -45) -> (10, -45)
  spline S71 degree 5 poles (10, -45) (11.9791, -46.0284) (15.9034, -48.1188) (21.6887, -51.3552) (29.1964, -55.8754) (38.2146, -61.8908) (46.833, -68.3041) (55.0184, -75.1487) (62.7516, -82.4437) (70.0489, -90.1727) (76.9426, -98.3036) (82.1609, -105.1037) (85.9183, -110.3595) (88.3548, -113.9314) (89.5561, -115.7344) knots 0 0 0 0 0 0 0.1 0.2 0.3 0.4 0.5 0.6 0.7 0.8 0.9 1 1 1 1 1 1
  arc A8 (89.5561, -115.7344) -> (117.3292, -90.3092) centre (108, -108) ccw
  spline S72 degree 5 poles (117.3292, -90.3092) (115.7178, -89.8787) (114.1172, -89.4373) (112.5273, -88.9851) (110.9483, -88.5219) (109.3801, -88.0477) knots -1 -1 -1 -1 -1 -1 -0.932954 -0.932954 -0.932954 -0.932954 -0.932954 -0.932954
  spline S73 degree 5 poles (109.3801, -88.0477) (108.6093, -87.8146) (105.5101, -86.8635) (100.1552, -85.1208) (92.6931, -82.436) (83.3647, -78.5649) (73.161, -73.5176) (63.577, -67.8424) (54.6474, -61.5042) (46.356, -54.5193) (38.6588, -46.9323) (32.9395, -40.4185) (28.8813, -35.2989) (26.2769, -31.7834) (25, -30) knots -0.932954 -0.932954 -0.932954 -0.932954 -0.932954 -0.932954 -0.9 -0.8 -0.7 -0.6 -0.5 -0.4 -0.3 -0.2 -0.1 0 0 0 0 0 0
  line L320 (25, -30) -> (25, 30)
  spline S74 degree 5 poles (25, 30) (26.2769, 31.7834) (28.8813, 35.2989) (32.9395, 40.4185) (38.6588, 46.9323) (46.356, 54.5193) (54.6474, 61.5042) (63.577, 67.8424) (73.161, 73.5176) (83.3647, 78.5649) (92.6931, 82.436) (100.1552, 85.1208) (105.5101, 86.8635) (108.6093, 87.8146) (109.3801, 88.0477) knots 0 0 0 0 0 0 0.1 0.2 0.3 0.4 0.5 0.6 0.7 0.8 0.9 0.932954 0.932954 0.932954 0.932954 0.932954 0.932954
  spline S75 degree 5 poles (109.3801, 88.0477) (110.9483, 88.5219) (112.5273, 88.9851) (114.1172, 89.4373) (115.7178, 89.8787) (117.3292, 90.3092) knots 0.932954 0.932954 0.932954 0.932954 0.932954 0.932954 1 1 1 1 1 1
  arc A9 (117.3292, 90.3092) -> (89.5561, 115.7344) centre (108, 108) ccw
  spline S76 degree 5 poles (89.5561, 115.7344) (88.3548, 113.9314) (85.9183, 110.3595) (82.1609, 105.1037) (76.9426, 98.3036) (70.0489, 90.1727) (62.7516, 82.4437) (55.0184, 75.1487) (46.833, 68.3041) (38.2146, 61.8908) (29.1964, 55.8754) (21.6887, 51.3552) (15.9034, 48.1188) (11.9791, 46.0284) (10, 45) knots -1 -1 -1 -1 -1 -1 -0.9 -0.8 -0.7 -0.6 -0.5 -0.4 -0.3 -0.2 -0.1 0 0 0 0 0 0
  line L321 (10, 45) -> (-10, 45)
  spline S77 degree 5 poles (-10, 45) (-11.9791, 46.0284) (-15.9034, 48.1188) (-21.6887, 51.3552) (-29.1964, 55.8754) (-38.2146, 61.8908) (-46.833, 68.3041) (-55.0184, 75.1487) (-62.7516, 82.4437) (-70.0489, 90.1727) (-76.9426, 98.3036) (-82.1609, 105.1037) (-85.9183, 110.3595) (-88.3548, 113.9314) (-89.5561, 115.7344) knots 0 0 0 0 0 0 0.1 0.2 0.3 0.4 0.5 0.6 0.7 0.8 0.9 1 1 1 1 1 1
  arc A10 (-89.5561, 115.7344) -> (-117.3292, 90.3092) centre (-108, 108) ccw
  spline S78 degree 5 poles (-117.3292, 90.3092) (-115.7178, 89.8787) (-114.1172, 89.4373) (-112.5273, 88.9851) (-110.9483, 88.5219) (-109.3801, 88.0477) knots -1 -1 -1 -1 -1 -1 -0.932954 -0.932954 -0.932954 -0.932954 -0.932954 -0.932954
  spline S79 degree 5 poles (-109.3801, 88.0477) (-108.6093, 87.8146) (-105.5101, 86.8635) (-100.1552, 85.1208) (-92.6931, 82.436) (-83.3647, 78.5649) (-73.161, 73.5176) (-63.577, 67.8424) (-54.6474, 61.5042) (-46.356, 54.5193) (-38.6588, 46.9323) (-32.9395, 40.4185) (-28.8813, 35.2989) (-26.2769, 31.7834) (-25, 30) knots -0.932954 -0.932954 -0.932954 -0.932954 -0.932954 -0.932954 -0.9 -0.8 -0.7 -0.6 -0.5 -0.4 -0.3 -0.2 -0.1 0 0 0 0 0 0
  line L322 (-25, 30) -> (-25, -30)
  spline S80 degree 5 poles (-25, -30) (-26.2769, -31.7834) (-28.8813, -35.2989) (-32.9395, -40.4185) (-38.6588, -46.9323) (-46.356, -54.5193) (-54.6474, -61.5042) (-63.577, -67.8424) (-73.161, -73.5176) (-83.3647, -78.5649) (-92.6931, -82.436) (-100.1552, -85.1208) (-105.5101, -86.8635) (-108.6093, -87.8146) (-109.3801, -88.0477) knots 0 0 0 0 0 0 0.1 0.2 0.3 0.4 0.5 0.6 0.7 0.8 0.9 0.932954 0.932954 0.932954 0.932954 0.932954 0.932954
  spline S81 degree 5 poles (-109.3801, -88.0477) (-110.9483, -88.5219) (-112.5273, -88.9851) (-114.1172, -89.4373) (-115.7178, -89.8787) (-117.3292, -90.3092) knots 0.932954 0.932954 0.932954 0.932954 0.932954 0.932954 1 1 1 1 1 1
  arc A11 (-117.3292, -90.3092) -> (-89.5561, -115.7344) centre (-108, -108) ccw
  spline S82 degree 5 poles (-89.5561, -115.7344) (-88.3548, -113.9314) (-85.9183, -110.3595) (-82.1609, -105.1037) (-76.9426, -98.3036) (-70.0489, -90.1727) (-62.7516, -82.4437) (-55.0184, -75.1487) (-46.833, -68.3041) (-38.2146, -61.8908) (-29.1964, -55.8754) (-21.6887, -51.3552) (-15.9034, -48.1188) (-11.9791, -46.0284) (-10, -45) knots -1 -1 -1 -1 -1 -1 -0.9 -0.8 -0.7 -0.6 -0.5 -0.4 -0.3 -0.2 -0.1 0 0 0 0 0 0
  circle A12 centre (17, -34) radius 2.5
  circle A13 centre (-17, -34) radius 2.5
  circle A14 centre (17, 34) radius 2.5
  circle A15 centre (-17, 34) radius 2.5
  line L323 (83.881, 103.9354) -> (86.9472, 94.7515)
  line L324 (86.9472, -94.7515) -> (83.881, -103.9354)
  line L325 (-83.881, -103.9354) -> (-86.9472, -94.7515)
sketch "Sketch13" plane through (0, 0, 6) normal (0, 0, 1) x (-1, 0, 0)
  line L0 (17, -31.5) -> (17, -36.5)
  arc A0 (17, -36.5) -> (17, -31.5) centre (17, -34) ccw
  line L1 (0, -2.5) -> (0, -20)
  arc A1 (-17, -31.5) -> (-17, -36.5) centre (-17, -34) ccw
  line L2 (-17, -31.5) -> (-17, -36.5)
  line L3 (-20, 0) -> (-2.5, 0)
  arc A2 (17, 31.5) -> (17, 36.5) centre (17, 34) ccw
  line L4 (17, 31.5) -> (17, 36.5)
  arc A3 (-17, 36.5) -> (-17, 31.5) centre (-17, 34) ccw
  line L5 (-17, 31.5) -> (-17, 36.5)
  dimension "d118" = 5
  constraint vertical L0
  constraint midpoint L0 A0.centre
  constraint symmetric L0.start L1 A1.start
  constraint symmetric L0.end L1 A1.end
  constraint symmetric A0 L1 A1
  constraint symmetric L0.start L3 A2.start
  constraint symmetric L0.end L3 A2.end
  constraint symmetric A0 L3 A2
  constraint symmetric A1.end L3 A3.start
  constraint symmetric A1.start L3 A3.end
  constraint symmetric A1 L3 A3
  measures "d118" diameter of A0
revolve "Revolve1" add sketch "Sketch13" angle 180 about axis through (-17, 31.5, 6) along (0, 1, 0) contours L0 A0 bodies 1
sketch "Sketch14" plane through (0, 0, 6) normal (0, 0, 1) x (-1, 0, 0)
  line L0 (-17, -36.5) -> (-17, -31.5)
  arc A0 (-17, -31.5) -> (-17, -36.5) centre (-17, -34) ccw
  line L1 (17, 31.5) -> (17, 36.5)
  arc A1 (17, 36.5) -> (17, 31.5) centre (17, 34) ccw
  line L2 (-17, 31.5) -> (-17, 36.5)
  arc A2 (-17, 36.5) -> (-17, 31.5) centre (-17, 34) ccw
  dimension "d120" = 5
  dimension "d121" = 5
  constraint vertical L0
  constraint midpoint L0 A0.centre
  constraint vertical L1
  constraint vertical L2
  measures "d120" diameter of A1
  measures "d121" diameter of A2
revolve "Revolve2" add sketch "Sketch14" angle 180 about axis through (17, -31.5, 6) along (0, -1, 0) contours L2 A2 bodies 1
revolve "Revolve3" add sketch "Sketch14" angle 180 about axis through (-17, -31.5, 6) along (0, -1, 0) contours L1 A1 bodies 1
revolve "Revolve4" add sketch "Sketch14" angle 180 about axis through (17, 31.5, 6) along (0, -1, 0) contours L0 A0 bodies 1
sketch "Sketch15" plane through (0, 0, -30) normal (0, 0, -1) x (1, 0, 0)
  line L0 (25, -50) -> (25, 50)
  line L1 (25, 50) -> (-25, 50)
  line L2 (-25, 50) -> (-25, -50)
  line L3 (-25, -50) -> (25, -50)
  line L4 (-17, 36.5) -> (-17, 31.5)
  arc A0 (-17, 31.5) -> (-17, 36.5) centre (-17, 34) ccw
  line L5 (0, -2.5) -> (0, -20)
  arc A1 (17, 36.5) -> (17, 31.5) centre (17, 34) ccw
  line L6 (17, 36.5) -> (17, 31.5)
  line L7 (20, 0) -> (2.5, 0)
  arc A2 (-17, -36.5) -> (-17, -31.5) centre (-17, -34) ccw
  line L8 (-17, -36.5) -> (-17, -31.5)
  arc A3 (17, -31.5) -> (17, -36.5) centre (17, -34) ccw
  line L9 (17, -36.5) -> (17, -31.5)
  dimension "d125" = 5
  constraint parallel L2 L4
  constraint midpoint L4 A0.centre
  constraint symmetric L4.start L5 A1.start
  constraint symmetric L4.end L5 A1.end
  constraint symmetric A0 L5 A1
  constraint symmetric L4.start L7 A2.start
  constraint symmetric L4.end L7 A2.end
  constraint symmetric A0 L7 A2
  constraint symmetric A1.end L7 A3.start
  constraint symmetric A1.start L7 A3.end
  constraint symmetric A1 L7 A3
  measures "d125" diameter of A0
revolve "Revolve5" add sketch "Sketch15" angle 180 about axis through (-17, -36.5, -30) along (0, 1, 0) contours L4 A0 bodies 1
revolve "Revolve6" add sketch "Sketch15" angle 180 about axis through (17, -36.5, -30) along (0, -1, 0) contours A1 L6 bodies 1
revolve "Revolve7" add sketch "Sketch15" angle 180 about axis through (-17, 36.5, -30) along (0, 1, 0) contours A2 L8 bodies 1
revolve "Revolve8" add sketch "Sketch15" angle 180 about axis through (17, 36.5, -30) along (0, -1, 0) contours A3 L9 bodies 1
sketch "Sketch17" plane through (0, 0, 6) normal (0, 0, 1) x (-1, 0, 0)
  circle A0 centre (108, -108) radius 3
  circle A1 centre (108, -100) radius 1.6
  circle A2 centre (116, -108) radius 1.6
  circle A3 centre (108, -116) radius 1.6
  circle A4 centre (100, -108) radius 1.6
  line L0 (0, -2.5) -> (0, -20)
  circle A5 centre (-100, -108) radius 1.6
  circle A6 centre (-108, -108) radius 3
  circle A7 centre (-108, -100) radius 1.6
  circle A8 centre (-116, -108) radius 1.6
  circle A9 centre (-108, -116) radius 1.6
  line L1 (-20, 0) -> (-2.5, 0)
  circle A10 centre (-100, 108) radius 1.6
  circle A11 centre (-116, 108) radius 1.6
  circle A12 centre (-108, 108) radius 3
  circle A13 centre (-108, 116) radius 1.6
  circle A14 centre (-108, 100) radius 1.6
  circle A15 centre (100, 108) radius 1.6
  circle A16 centre (116, 108) radius 1.6
  circle A17 centre (108, 108) radius 3
  circle A18 centre (108, 100) radius 1.6
  circle A19 centre (108, 116) radius 1.6
  point P0 (108, -108)
  point P1 (108, 108)
  dimension "d146" = 6
  dimension "d147" = 3.2
  dimension "d148" = 3.2
  dimension "d149" = 3.2
  dimension "d150" = 3.2
  dimension "d151" = 8
  dimension "d152" = 8
  dimension "d153" = 8
  dimension "d154" = 8
  constraint coincident P0 A0.centre
  constraint symmetric A0 L0 A6
  constraint symmetric A1 L0 A7
  constraint symmetric A2 L0 A8
  constraint symmetric A3 L0 A9
  constraint symmetric A4 L0 A5
  constraint symmetric P0 L1 A17.centre
  constraint symmetric A0 L1 A17
  constraint symmetric A1 L1 A18
  constraint symmetric A2 L1 A16
  constraint symmetric A3 L1 A19
  constraint symmetric A4 L1 A15
  constraint symmetric A5 L1 A10
  constraint symmetric A6 L1 A12
  constraint symmetric A7 L1 A14
  constraint symmetric A8 L1 A11
  constraint symmetric A9 L1 A13
  measures "d146" diameter of A0
  measures "d147" diameter of A1
  measures "d148" diameter of A2
  measures "d149" diameter of A3
  measures "d150" diameter of A4
  measures "d151" distance of P0 A1.centre
  measures "d152" distance of P0 A2.centre
  measures "d153" distance of P0 A3.centre
  measures "d154" distance of P0 A4.centre
extrude "Extrude16" cut sketch "Sketch17" against normal blind 19 contours A0 | A1 | A2 | A3 | A4 bodies 1
sketch "Sketch18" plane through (0, 0, 6) normal (0, 0, 1) x (-1, 0, 0)
  circle A0 centre (108, -108) radius 17
  line L0 (0, -2.5) -> (0, -20)
  circle A1 centre (-108, -108) radius 17
  line L1 (-20, 0) -> (-2.5, 0)
  circle A2 centre (-108, 108) radius 17
  circle A3 centre (108, 108) radius 17
  dimension "d157" = 34
  constraint symmetric A0 L0 A1
  constraint symmetric A0 L1 A3
  constraint symmetric A1 L1 A2
  measures "d157" diameter of A0
extrude "Extrude17" cut sketch "Sketch18" against normal blind 1 contours A0 bodies 1
extrude "Extrude18" cut sketch "Sketch17" against normal blind 16 contours A15 | A16 | A17 | A18 | A19 bodies 1
extrude "Extrude19" cut sketch "Sketch17" against normal blind 12 contours A10 | A11 | A12 | A13 | A14 bodies 1
extrude "Extrude20" cut sketch "Sketch17" against normal blind 14 contours A5 | A6 | A7 | A8 | A9 bodies 1
extrude "Extrude21" cut sketch "Sketch18" against normal blind 1 contours A3 bodies 1
extrude "Extrude22" cut sketch "Sketch18" against normal blind 1 contours A2 bodies 1
extrude "Extrude23" cut sketch "Sketch18" against normal blind 1 contours A1 bodies 1
extrude "Extrude24" cut sketch "Sketch5" against normal blind 10 contours A2 | A3 | A4 | A5 bodies 1
extrude "Extrude25" cut sketch "Sketch5" against normal blind 10 contours L428 S12 L471 L519 bodies 1
